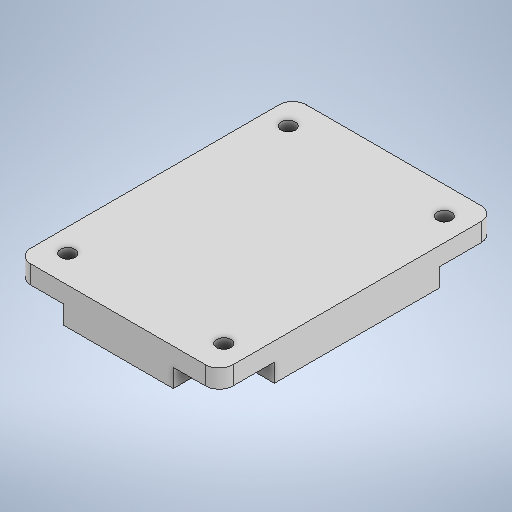
# Autodesk Inventor part: motor_driver_support
Saved by Autodesk Inventor 2026.1 (Build 301233000, 233)
## iProperties
Created: 2025-09-28
Part Number: motor_driver_support
Material: Generic
Document SubType Name: Modeling
Designer: chris
Density: 1 g/cm^3
Appearance: Default
Author: chris
Autodesk Inventor part; units mm, degrees
ref_plane "YZ Plane" through (0, 0, 0) normal (1, 0, 0) x (0, 1, 0)
ref_plane "XZ Plane" through (0, 0, 0) normal (0, 1, 0) x (-1, 0, 0)
ref_plane "XY Plane" through (0, 0, 0) normal (0, 0, 1) x (1, 0, 0)
sketch "Sketch1" plane through (0, 0, 0) normal (0, 1, 0) x (-1, 0, 0)
  line L0 (22, 30) -> (-22, 30)
  line L1 (-22, 30) -> (-22, -30)
  line L2 (-22, -30) -> (22, -30)
  line L3 (22, -30) -> (22, 30)
  line L4 (22, 30) -> (-22, -30) construction
  line L5 (-22, 30) -> (22, -30) construction
  point P0 (0, 0)
  dimension "d0" = 44
  dimension "d1" = 60
  constraints: 12 end point, 2 midpoint, 2 parallel, 1 horizontal, 1 perpendicular
  measures "d0" distance of L2.end L1.end
  measures "d1" distance of L1.end L0.end
extrude "Extrusion1" add sketch "Sketch1" along normal blind 8
sketch "Sketch4" plane through (0, 8, 0) normal (0, 1, 0) x (1, 0, 0)
  circle A0 centre (-17, -24) radius 1.55
  circle A1 centre (17, 24) radius 1.55
  circle A2 centre (17, -24) radius 1.55
  circle A3 centre (-17, 24) radius 1.55
  point P0 (0, 0)
  dimension "d6" = 3.1
  dimension "d7" = 3.1
  dimension "d8" = 3.1
  dimension "d9" = 3.1
  dimension "d10" = 17
  dimension "d11" = 24
  dimension "d12" = 17
  dimension "d13" = 17
  dimension "d14" = 17
  dimension "d15" = 24
  dimension "d16" = 24
  dimension "d17" = 24
  constraints: 4 centre point
  measures "d6" diameter of A0
  measures "d7" diameter of A1
  measures "d8" diameter of A2
  measures "d9" diameter of A3
  measures "d10" horizontal distance of A0.centre point (0, 0)
  measures "d11" vertical distance of A0.centre point (0, 0)
  measures "d12" horizontal distance of A3.centre point (0, 0)
  measures "d13" horizontal distance of A1.centre point (0, 0)
  measures "d14" horizontal distance of point (0, 0) A2.centre
  measures "d15" vertical distance of point (0, 0) A2.centre
  measures "d16" vertical distance of point (0, 0) A1.centre
  measures "d17" vertical distance of A3.centre point (0, 0)
hole "Hole1" at (-17, 8, 24) at (-17, 8, -24) at (17, 8, -24) at (17, 8, 24) direction (0, -1, 0) diameter 3.1 depth 8 tip angle 118
sketch "Sketch5" plane through (0, 0, 0) normal (0, -1, 0) x (1, 0, 0)
  line L0 (-12, -18) -> (-22, -18)
  line L1 (-22, -18) -> (-22, -30)
  line L2 (-22, -30) -> (-12, -30)
  line L3 (-12, -30) -> (-12, -18)
  line L4 (22, -18) -> (12, -18)
  line L5 (12, -18) -> (12, -30)
  line L6 (12, -30) -> (22, -30)
  line L7 (22, -30) -> (22, -18)
  line L8 (22, 30) -> (12, 30)
  line L9 (12, 30) -> (12, 18)
  line L10 (12, 18) -> (22, 18)
  line L11 (22, 18) -> (22, 30)
  line L12 (-12, 30) -> (-22, 30)
  line L13 (-22, 30) -> (-22, 18)
  line L14 (-22, 18) -> (-12, 18)
  line L15 (-12, 18) -> (-12, 30)
  line L16 (-22, -30) -> (-22, 30) projected
  line L17 (22, -30) -> (-22, -30) projected
  line L18 (22, 30) -> (22, -30) projected
  line L19 (-22, 30) -> (22, 30) projected
  point P0 (0, 0)
  dimension "d25" = 10
  dimension "d26" = 12
  dimension "d27" = 10
  dimension "d28" = 12
  dimension "d29" = 10
  dimension "d30" = 12
  dimension "d31" = 10
  dimension "d32" = 12
  constraints: 32 end point, 8 collinear, 8 parallel, 4 horizontal, 4 perpendicular
  measures "d25" distance of L2.end L1.end
  measures "d26" distance of L1.end L0.end
  measures "d27" distance of L6.end L5.end
  measures "d28" distance of L5.end L4.end
  measures "d29" distance of L10.end L9.end
  measures "d30" distance of L9.end L8.end
  measures "d31" distance of L14.end L13.end
  measures "d32" distance of L13.end L12.end
extrude "Extrusion2" cut sketch "Sketch5" against normal blind 4 contours L3 L2 L1 L0 | L13 L12 L15 L14 | L5 L4 L7 L6 | L8 L11 L10 L9
fillet "Fillet1" radius 3 4 edges at (22, 6, -30) (-22, 6, -30) (22, 6, 30) (-22, 6, 30)
equation "\"d12\" = d10"
equation "\"d13\" = d10"
equation "\"d14\" = d10"
equation "\"d15\" = d11"
equation "\"d16\" = d11"
equation "\"d17\" = d11"
equation "\"d27\" = d25"
equation "\"d28\" = d26"
equation "\"d29\" = d25"
equation "\"d30\" = d26"
equation "\"d31\" = d25"
equation "\"d32\" = d26"
body "Solid1"
